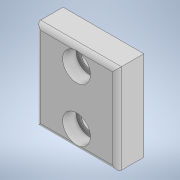
# Autodesk Inventor part: ChassisLegV1
Saved by Autodesk Inventor 2020 (Build 240168000, 168)
## iProperties
Created: 2023-02-16
Part Number: ChassisLegV1
Material: Generic
Document SubType Name: Modeling
Designer: agraa4529
Density: 1 g/cm^3
Appearance: Default
Author: agraa4529
Autodesk Inventor part; units mm, degrees
ref_plane "YZ Plane" through (0, 0, 0) normal (1, 0, 0) x (0, 1, 0)
ref_plane "XZ Plane" through (0, 0, 0) normal (0, 1, 0) x (-1, 0, 0)
ref_plane "XY Plane" through (0, 0, 0) normal (0, 0, 1) x (1, 0, 0)
sketch "Sketch1" plane through (0, 0, 0) normal (0, 0, 1) x (1, 0, 0)
  line L0 (-9, 10) -> (9, 10)
  line L1 (9, 10) -> (9, -10)
  line L2 (9, -10) -> (-9, -10)
  line L3 (-9, -10) -> (-9, 10)
  line L4 (-9, 10) -> (9, -10) construction
  line L5 (9, 10) -> (-9, -10) construction
  line L6 (0, 0) -> (0, 6)
  line L7 (0, 0) -> (0, -6)
  circle A0 centre (0, 6) radius 1.9
  circle A1 centre (0, -6) radius 1.9
  dimension "d0" = 18
  dimension "d1" = 20
  dimension "d2" = 6
  dimension "d3" = 6
  dimension "d4" = 3.8
  dimension "d5" = 3.8
  constraints: 16 end point, 2 centre point, 2 coincident, 2 midpoint, 2 parallel, 2 vertical, 1 horizontal, 1 perpendicular
  measures "d0" distance of L1.end L2.end
  measures "d1" distance of L0.end L1.end
  measures "d2" distance of L6.start L6.end
  measures "d3" distance of L6.start L7.end
  measures "d4" diameter of A0
  measures "d5" diameter of A1
extrude "Extrusion1" add sketch "Sketch1" along normal blind 6
sketch "Sketch2" plane through (0, 0, 6) normal (0, 0, 1) x (1, 0, 0)
  circle A0 centre (0, 6) radius 1.9 projected
  circle A1 centre (0, 6) radius 3.1
  circle A2 centre (0, -6) radius 1.9 projected
  circle A3 centre (0, -6) radius 3.1
  point P0 (0, 0)
  dimension "d8" = 6.2
  dimension "d9" = 6.2
  constraints: 2 centre point, 2 coincident
  measures "d8" diameter of A1
  measures "d9" diameter of A3
extrude "Extrusion2" cut sketch "Sketch2" against normal blind 3
fillet "Fillet1" radius 1 4 edges at (0, 10, 6) (-9, 0, 6) (0, -10, 6) (9, 0, 6)
body "Solid1"
